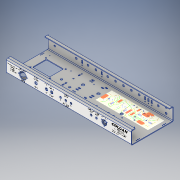
# Autodesk Inventor part: mainChassis
Saved by Autodesk Inventor 2018.1 (Build 221171000, 171)
## iProperties
Created: 2019-02-19
Part Number: mainChassis
Material: Aluminum 6061
Document SubType Name: Sheet Metal
Designer: RCCol
Density: 2.7 g/cm^3
Sheet Metal Rule: .125 thick aluminum
Appearance: Aluminum - Flat
Flat Pattern Width: 34.7497 cm
Flat Pattern Length: 60.325 cm
Flat Pattern Area: 2096.27 cm^2
Sheet Metal Width: 13.681 in
Sheet Metal Length: 23.750 in
Sheet Metal Area: 324.923 in^2
Author: RCCol
Autodesk Inventor part; units mm, degrees
ref_plane "YZ Plane" through (0, 0, 0) normal (1, 0, 0) x (0, 1, 0)
ref_plane "XZ Plane" through (0, 0, 0) normal (0, 1, 0) x (-1, 0, 0)
ref_plane "XY Plane" through (0, 0, 0) normal (0, 0, 1) x (1, 0, 0)
sketch "Sketch1" plane through (0, 0, 0) normal (0, 1, 0) x (-1, 0, 0)
  line L0 (0, 0) -> (-603.25, 0)
  line L1 (-603.25, 0) -> (-603.25, -204.47)
  line L2 (-603.25, -204.47) -> (0, -204.47)
  line L3 (0, -204.47) -> (0, 0)
  line L4 (0, 0) -> (-254, 0)
  line L5 (0, -79.375) -> (0, 0)
  dimension "d0" = 603.25
  dimension "d1" = 204.47
  constraints: 12 end point, 2 horizontal, 2 parallel, 1 perpendicular
  measures "d0" distance of L2.end L1.end
  measures "d1" distance of L1.end L0.end
extrude "Plate1" add sketch "Sketch1" along normal blind 3.175
sketch "Sketch2" plane through (0, 3.175, 0) normal (0, 1, 0) x (1, 0, 0)
  line L0 (41.3, 154.94) -> (117.45, 154.94)
  arc A0 (120.65, 151.74) -> (117.45, 154.94) centre (117.45, 151.74) ccw
  line L1 (41.3, 87.63) -> (117.45, 87.63)
  arc A1 (117.45, 87.63) -> (120.65, 90.83) centre (117.45, 90.83) ccw
  line L2 (38.1, 151.74) -> (38.1, 90.83)
  arc A2 (41.3, 154.94) -> (38.1, 151.74) centre (41.3, 151.74) ccw
  arc A3 (38.1, 90.83) -> (41.3, 87.63) centre (41.3, 90.83) ccw
  circle A4 centre (31.75, 177.5295) radius 1.5
  line L3 (120.65, 151.74) -> (120.65, 90.83)
  circle A5 centre (147.375, 75.2475) radius 1.65
  circle A6 centre (147.375, 164.1475) radius 1.65
  circle A7 centre (185.1575, 138.7475) radius 2.65
  circle A8 centre (185.1575, 178.435) radius 2.65
  circle A9 centre (235.9575, 87.1648) radius 2.65
  circle A10 centre (243.895, 87.1648) radius 2.65
  circle A11 centre (235.9575, 169.7148) radius 2.65
  circle A12 centre (243.895, 169.7148) radius 2.65
  circle A13 centre (259.135, 75.2475) radius 1.65
  circle A14 centre (355.6, 82.2325) radius 1.65
  circle A15 centre (259.135, 164.1475) radius 1.65
  circle A16 centre (355.6, 139.3825) radius 1.65
  circle A17 centre (536.575, 82.2325) radius 1.65
  circle A18 centre (536.575, 139.3825) radius 1.65
  arc A19 (187.6575, 169.4256) -> (182.6575, 169.4256) centre (185.1575, 169.4256) ccw
  arc A20 (182.6575, 164.4256) -> (187.6575, 164.4256) centre (185.1575, 164.4256) ccw
  line L4 (187.6575, 169.4256) -> (187.6575, 164.4256)
  line L5 (182.6575, 169.4256) -> (182.6575, 164.4256)
  arc A21 (187.6575, 90.4475) -> (182.6575, 90.4475) centre (185.1575, 90.4475) ccw
  arc A22 (182.6575, 85.4475) -> (187.6575, 85.4475) centre (185.1575, 85.4475) ccw
  line L6 (187.6575, 90.4475) -> (187.6575, 85.4475)
  line L7 (182.6575, 90.4475) -> (182.6575, 85.4475)
  arc A23 (308.1355, 175.935) -> (308.1355, 180.935) centre (308.1355, 178.435) ccw
  arc A24 (301.1355, 180.935) -> (301.1355, 175.935) centre (301.1355, 178.435) ccw
  line L8 (308.1355, 175.935) -> (301.1355, 175.935)
  line L9 (308.1355, 180.935) -> (301.1355, 180.935)
  arc A25 (243.048, 175.935) -> (243.048, 180.935) centre (243.048, 178.435) ccw
  arc A26 (236.048, 180.935) -> (236.048, 175.935) centre (236.048, 178.435) ccw
  line L10 (243.048, 175.935) -> (236.048, 175.935)
  line L11 (243.048, 180.935) -> (236.048, 180.935)
  arc A27 (298.195, 167.2148) -> (298.195, 172.2148) centre (298.195, 169.7148) ccw
  arc A28 (291.195, 172.2148) -> (291.195, 167.2148) centre (291.195, 169.7148) ccw
  line L12 (298.195, 167.2148) -> (291.195, 167.2148)
  line L13 (298.195, 172.2148) -> (291.195, 172.2148)
  arc A29 (308.1355, 110.435) -> (308.1355, 115.435) centre (308.1355, 112.935) ccw
  arc A30 (301.1355, 115.435) -> (301.1355, 110.435) centre (301.1355, 112.935) ccw
  line L14 (308.1355, 110.435) -> (301.1355, 110.435)
  line L15 (308.1355, 115.435) -> (301.1355, 115.435)
  arc A31 (308.1355, 99.735) -> (308.1355, 104.735) centre (308.1355, 102.235) ccw
  arc A32 (301.1355, 104.735) -> (301.1355, 99.735) centre (301.1355, 102.235) ccw
  line L16 (308.1355, 99.735) -> (301.1355, 99.735)
  line L17 (308.1355, 104.735) -> (301.1355, 104.735)
  arc A33 (243.048, 110.435) -> (243.048, 115.435) centre (243.048, 112.935) ccw
  arc A34 (236.048, 115.435) -> (236.048, 110.435) centre (236.048, 112.935) ccw
  line L18 (243.048, 110.435) -> (236.048, 110.435)
  line L19 (243.048, 115.435) -> (236.048, 115.435)
  arc A35 (243.048, 99.735) -> (243.048, 104.735) centre (243.048, 102.235) ccw
  arc A36 (236.048, 104.735) -> (236.048, 99.735) centre (236.048, 102.235) ccw
  line L20 (243.048, 99.735) -> (236.048, 99.735)
  line L21 (243.048, 104.735) -> (236.048, 104.735)
  arc A37 (298.195, 84.6648) -> (298.195, 89.6648) centre (298.195, 87.1648) ccw
  arc A38 (291.195, 89.6648) -> (291.195, 84.6648) centre (291.195, 87.1648) ccw
  line L22 (298.195, 84.6648) -> (291.195, 84.6648)
  line L23 (298.195, 89.6648) -> (291.195, 89.6648)
  circle A39 centre (237.6, 35.56) radius 15.1
  arc A40 (239.251, 57.4158) -> (238.6557, 58.0111) centre (238.6557, 57.4158) ccw
  arc A41 (238.6557, 53.1089) -> (239.251, 53.7042) centre (238.6557, 53.7042) ccw
  line L24 (239.251, 53.7042) -> (239.251, 57.4158)
  arc A42 (236.5443, 58.0111) -> (235.949, 57.4158) centre (236.5443, 57.4158) ccw
  line L25 (235.949, 53.7042) -> (235.949, 57.4158)
  line L26 (238.6557, 58.0111) -> (236.5443, 58.0111)
  line L27 (238.6557, 53.1089) -> (236.5443, 53.1089)
  arc A43 (235.949, 53.7042) -> (236.5443, 53.1089) centre (236.5443, 53.7042) ccw
  arc A44 (239.251, 17.4158) -> (238.6557, 18.0111) centre (238.6557, 17.4158) ccw
  arc A45 (238.6557, 13.1089) -> (239.251, 13.7042) centre (238.6557, 13.7042) ccw
  line L28 (239.251, 13.7042) -> (239.251, 17.4158)
  arc A46 (236.5443, 18.0111) -> (235.949, 17.4158) centre (236.5443, 17.4158) ccw
  line L29 (235.949, 13.7042) -> (235.949, 17.4158)
  line L30 (238.6557, 18.0111) -> (236.5443, 18.0111)
  line L31 (238.6557, 13.1089) -> (236.5443, 13.1089)
  arc A47 (235.949, 13.7042) -> (236.5443, 13.1089) centre (236.5443, 13.7042) ccw
  circle A48 centre (174.1, 35.56) radius 15.1
  arc A49 (175.751, 57.4158) -> (175.1557, 58.0111) centre (175.1557, 57.4158) ccw
  arc A50 (175.1557, 53.1089) -> (175.751, 53.7042) centre (175.1557, 53.7042) ccw
  line L32 (175.751, 53.7042) -> (175.751, 57.4158)
  arc A51 (173.0443, 58.0111) -> (172.449, 57.4158) centre (173.0443, 57.4158) ccw
  line L33 (172.449, 53.7042) -> (172.449, 57.4158)
  line L34 (175.1557, 58.0111) -> (173.0443, 58.0111)
  line L35 (175.1557, 53.1089) -> (173.0443, 53.1089)
  arc A52 (172.449, 53.7042) -> (173.0443, 53.1089) centre (173.0443, 53.7042) ccw
  arc A53 (175.751, 17.4158) -> (175.1557, 18.0111) centre (175.1557, 17.4158) ccw
  arc A54 (175.1557, 13.1089) -> (175.751, 13.7042) centre (175.1557, 13.7042) ccw
  line L36 (175.751, 13.7042) -> (175.751, 17.4158)
  arc A55 (173.0443, 18.0111) -> (172.449, 17.4158) centre (173.0443, 17.4158) ccw
  line L37 (172.449, 13.7042) -> (172.449, 17.4158)
  line L38 (175.1557, 18.0111) -> (173.0443, 18.0111)
  line L39 (175.1557, 13.1089) -> (173.0443, 13.1089)
  arc A56 (172.449, 13.7042) -> (173.0443, 13.1089) centre (173.0443, 13.7042) ccw
  circle A57 centre (110.6, 35.56) radius 15.1
  arc A58 (112.251, 57.4158) -> (111.6557, 58.0111) centre (111.6557, 57.4158) ccw
  arc A59 (111.6557, 53.1089) -> (112.251, 53.7042) centre (111.6557, 53.7042) ccw
  line L40 (112.251, 53.7042) -> (112.251, 57.4158)
  arc A60 (109.5443, 58.0111) -> (108.949, 57.4158) centre (109.5443, 57.4158) ccw
  line L41 (108.949, 53.7042) -> (108.949, 57.4158)
  line L42 (111.6557, 58.0111) -> (109.5443, 58.0111)
  line L43 (111.6557, 53.1089) -> (109.5443, 53.1089)
  arc A61 (108.949, 53.7042) -> (109.5443, 53.1089) centre (109.5443, 53.7042) ccw
  arc A62 (112.251, 17.4158) -> (111.6557, 18.0111) centre (111.6557, 17.4158) ccw
  arc A63 (111.6557, 13.1089) -> (112.251, 13.7042) centre (111.6557, 13.7042) ccw
  line L44 (112.251, 13.7042) -> (112.251, 17.4158)
  arc A64 (109.5443, 18.0111) -> (108.949, 17.4158) centre (109.5443, 17.4158) ccw
  line L45 (108.949, 13.7042) -> (108.949, 17.4158)
  line L46 (111.6557, 18.0111) -> (109.5443, 18.0111)
  line L47 (111.6557, 13.1089) -> (109.5443, 13.1089)
  arc A65 (108.949, 13.7042) -> (109.5443, 13.1089) centre (109.5443, 13.7042) ccw
  circle A66 centre (47.1, 35.56) radius 15.1
  arc A67 (48.751, 57.4158) -> (48.1557, 58.0111) centre (48.1557, 57.4158) ccw
  arc A68 (48.1557, 53.1089) -> (48.751, 53.7042) centre (48.1557, 53.7042) ccw
  line L48 (48.751, 53.7042) -> (48.751, 57.4158)
  arc A69 (46.0443, 58.0111) -> (45.449, 57.4158) centre (46.0443, 57.4158) ccw
  line L49 (45.449, 53.7042) -> (45.449, 57.4158)
  line L50 (48.1557, 58.0111) -> (46.0443, 58.0111)
  line L51 (48.1557, 53.1089) -> (46.0443, 53.1089)
  arc A70 (45.449, 53.7042) -> (46.0443, 53.1089) centre (46.0443, 53.7042) ccw
  arc A71 (48.751, 17.4158) -> (48.1557, 18.0111) centre (48.1557, 17.4158) ccw
  arc A72 (48.1557, 13.1089) -> (48.751, 13.7042) centre (48.1557, 13.7042) ccw
  line L52 (48.751, 13.7042) -> (48.751, 17.4158)
  arc A73 (46.0443, 18.0111) -> (45.449, 17.4158) centre (46.0443, 17.4158) ccw
  line L53 (45.449, 13.7042) -> (45.449, 17.4158)
  line L54 (48.1557, 18.0111) -> (46.0443, 18.0111)
  line L55 (48.1557, 13.1089) -> (46.0443, 13.1089)
  arc A74 (45.449, 13.7042) -> (46.0443, 13.1089) centre (46.0443, 13.7042) ccw
  circle A75 centre (159.7575, 106.3403) radius 4.8
  circle A76 centre (212.2, 93.5148) radius 4.8
  circle A77 centre (309.5568, 135.335) radius 6.35
  circle A78 centre (234.6268, 135.335) radius 6.35
  circle A79 centre (269.35, 26.9408) radius 1.651
  circle A80 centre (501.65, 37.1475) radius 9.525
  circle A81 centre (491.5472, 47.2503) radius 1.651
  circle A82 centre (511.7528, 27.0447) radius 1.651
  circle A83 centre (444.5, 37.1475) radius 9.525
  circle A84 centre (434.3972, 47.2503) radius 1.651
  circle A85 centre (454.6028, 27.0447) radius 1.651
  circle A86 centre (406.4, 37.1475) radius 9.525
  circle A87 centre (396.2972, 47.2503) radius 1.651
  circle A88 centre (416.5028, 27.0447) radius 1.651
  circle A89 centre (368.3, 37.1475) radius 9.525
  circle A90 centre (358.1972, 47.2503) radius 1.651
  circle A91 centre (378.4028, 27.0447) radius 1.651
  circle A92 centre (330.2, 37.1475) radius 9.525
  circle A93 centre (320.0972, 47.2503) radius 1.651
  circle A94 centre (340.3028, 27.0447) radius 1.651
  circle A95 centre (205.85, 26.9408) radius 1.651
  circle A96 centre (78.85, 26.9408) radius 1.651
  circle A97 centre (78.85, 63.0879) radius 1.651
  circle A98 centre (19.05, 63.0879) radius 1.651
  circle A99 centre (503.2375, 162.56) radius 1.651
  circle A100 centre (142.35, 26.035) radius 1.651
  circle A101 centre (22.225, 20.5908) radius 1.651
  arc A102 (187.6575, 104.4569) -> (182.6575, 104.4569) centre (185.1575, 104.4569) ccw
  arc A103 (182.6575, 99.4569) -> (187.6575, 99.4569) centre (185.1575, 99.4569) ccw
  line L56 (187.6575, 104.4569) -> (187.6575, 99.4569)
  line L57 (182.6575, 104.4569) -> (182.6575, 99.4569)
  circle A104 centre (458.7875, 172.085) radius 1.651
  circle A105 centre (193.85, 60.5908) radius 1.65
  circle A106 centre (217.85, 60.5908) radius 1.65
  circle A107 centre (205.85, 60.5908) radius 4.826
  circle A108 centre (257.35, 59.0033) radius 1.65
  circle A109 centre (281.35, 59.0033) radius 1.65
  circle A110 centre (269.35, 59.0033) radius 4.826
  circle A111 centre (137.16, 62.3578) radius 1.651
  circle A112 centre (522.2875, 162.56) radius 1.651
  circle A113 centre (477.8375, 172.085) radius 1.651
  circle A114 centre (491.2375, 172.085) radius 1.651
  circle A115 centre (445.3875, 172.085) radius 1.651
  circle A116 centre (438.15, 78.2625) radius 4.826
  circle A117 centre (412.75, 78.2625) radius 4.826
  circle A118 centre (467.3028, 92.3925) radius 2.3813
  circle A119 centre (506.908, 112.5724) radius 2.3813
  circle A120 centre (449.8015, 107.4686) radius 6.35
  circle A121 centre (494.6689, 127.4196) radius 2.3813
  circle A122 centre (368.3, 21.2725) radius 1.651
  circle A123 centre (501.65, 53.0225) radius 1.651
  circle A124 centre (406.4, 53.0225) radius 1.651
  circle A125 centre (368.3, 53.0225) radius 1.651
  circle A126 centre (31.75, 159.385) radius 3.175
  circle A127 centre (127, 159.385) radius 3.175
  circle A128 centre (31.75, 83.185) radius 3.175
  circle A129 centre (127, 83.185) radius 3.175
  circle A130 centre (539.75, 37.1475) radius 9.525
  circle A131 centre (529.6472, 47.2503) radius 1.651
  circle A132 centre (549.8528, 27.0447) radius 1.651
  circle A133 centre (539.75, 53.0225) radius 1.651
  circle A134 centre (78.85, 35.56) radius 3.2385
  circle A135 centre (142.35, 35.56) radius 3.2385
  circle A136 centre (205.85, 35.56) radius 3.2385
  circle A137 centre (269.35, 35.56) radius 3.2385
  circle A138 centre (6.35, 165.735) radius 2.667
  circle A139 centre (6.35, 158.3944) radius 1.5875
  circle A140 centre (6.35, 173.0756) radius 1.5875
  circle A141 centre (6.35, 38.735) radius 2.667
  circle A142 centre (6.35, 31.3944) radius 1.5875
  circle A143 centre (6.35, 46.0756) radius 1.5875
  circle A144 centre (596.9, 38.735) radius 2.667
  circle A145 centre (596.9, 46.0756) radius 1.5875
  circle A146 centre (596.9, 31.3944) radius 1.5875
  circle A147 centre (596.9, 165.735) radius 2.667
  circle A148 centre (596.9, 173.0756) radius 1.5875
  circle A149 centre (596.9, 158.3944) radius 1.5875
  circle A150 centre (288.4, 35.56) radius 3.2385
  circle A151 centre (117.45, 90.83) radius 3.2
  circle A152 centre (41.3, 90.83) radius 3.2
  circle A153 centre (41.3, 151.74) radius 3.2
  circle A154 centre (117.45, 151.74) radius 3.2
  line L58 (117.45, 87.63) -> (41.3, 87.63)
  line L59 (41.3, 87.63) -> (41.3, 154.94)
  line L60 (41.3, 154.94) -> (117.45, 154.94)
  line L61 (117.45, 154.94) -> (117.45, 87.63)
  line L62 (38.1, 90.83) -> (120.65, 90.83)
  line L63 (120.65, 90.83) -> (120.65, 151.74)
  line L64 (120.65, 151.74) -> (38.1, 151.74)
  line L65 (38.1, 151.74) -> (38.1, 90.83)
  constraints: 153 centre point, 132 end point, 116 point on circle, 4 coincident, 4 parallel, 2 horizontal, 2 horizontal alignment, 2 perpendicular, 2 point on line, 4 other
extrude "Cut1" cut sketch "Sketch2" against normal blind 3.175
sketch "Sketch3" plane through (603.25, 0, -3.175) normal (0, 0, 1) x (1, 0, 0)
  line L0 (-603.25, 0) -> (0, 0)
  line L1 (0, 0) -> (0, 63.5)
  line L2 (0, 63.5) -> (-603.25, 63.5)
  line L3 (-603.25, 63.5) -> (-603.25, 0)
  constraints: 6 end point, 1 horizontal, 1 perpendicular, 1 vertical
edge flange "Flange1" height 63.5 angle 90 thickness 3.175 bend radius 3.175 thickness toward (0, 0, 1) relief straight relief width 3.175 relief depth 1.5875 edges at (301.625, 3.175, 0) wall of the first edge with corners at (0, 0, -3.175) (603.25, 0, -3.175) (603.25, 63.5, -3.175) (0, 63.5, -3.175)
bend "Bend1"
corner "Corner1"
sketch "Sketch4" plane through (603.25, 60.325, 0) normal (0, 1, 0) x (-1, 0, 0)
  line L0 (603.25, 0) -> (0, 0)
  line L1 (0, 0) -> (0, -19.05)
  line L2 (0, -19.05) -> (603.25, -19.05)
  line L3 (603.25, -19.05) -> (603.25, 0)
  constraints: 6 end point, 1 horizontal, 1 perpendicular, 1 vertical
edge flange "Flange2" height 19.05 angle 90 thickness 3.175 bend radius 3.175 thickness toward (0, 1, 0) relief straight relief width 3.175 relief depth 1.5875 edges at (301.625, 63.5, -3.175) wall of the first edge with corners at (0, 60.325, 0) (603.25, 60.325, 0) (603.25, 60.325, -19.05) (0, 60.325, -19.05)
bend "Bend2"
corner "Corner2"
sketch "Sketch5" plane through (0, 6.35, 0) normal (0, 0, 1) x (1, 0, 0)
  circle A0 centre (78.85, 25.4) radius 17.4625
  circle A1 centre (99.805, 25.4) radius 1.778
  circle A2 centre (57.895, 25.4) radius 1.778
  line L0 (148.065, 22.0907) -> (148.065, 28.7093)
  line L1 (136.635, 22.0907) -> (136.635, 28.7093)
  arc A3 (136.635, 22.0907) -> (148.065, 22.0907) centre (142.35, 25.4) ccw
  arc A4 (148.065, 28.7093) -> (136.635, 28.7093) centre (142.35, 25.4) ccw
  line L2 (193.9018, 20.2386) -> (192.3982, 20.2386)
  arc A5 (193.9018, 19.2226) -> (192.3982, 19.2226) centre (193.15, 25.4) ccw
  line L3 (192.3982, 20.2386) -> (192.3982, 19.2226)
  line L4 (193.9018, 19.2226) -> (193.9018, 20.2386)
  line L5 (219.3018, 20.2386) -> (217.7982, 20.2386)
  arc A6 (219.3018, 19.2226) -> (217.7982, 19.2226) centre (218.55, 25.4) ccw
  line L6 (217.7982, 20.2386) -> (217.7982, 19.2226)
  line L7 (219.3018, 19.2226) -> (219.3018, 20.2386)
  circle A7 centre (261.3213, 25.4) radius 4.7625
  circle A8 centre (286.7213, 25.4) radius 4.7625
  circle A9 centre (312.1213, 25.4) radius 4.7625
  circle A10 centre (409.575, 25.5399) radius 4.7625
  circle A11 centre (434.975, 25.5399) radius 4.7625
  circle A12 centre (473.075, 25.5399) radius 12.1031
  circle A13 centre (460.2734, 32.9821) radius 1.778
  circle A14 centre (485.8766, 32.9821) radius 1.778
  circle A15 centre (473.075, 10.7317) radius 1.778
  line L8 (136.635, 28.7093) -> (148.065, 28.7093)
  line L9 (148.065, 28.7093) -> (148.065, 22.0907)
  line L10 (148.065, 22.0907) -> (136.635, 22.0907)
  line L11 (136.635, 22.0907) -> (136.635, 28.7093)
  arc A16 (148.065, 28.7093) -> (136.635, 28.7093) centre (142.35, 25.4) ccw
  arc A17 (136.635, 22.0907) -> (148.065, 22.0907) centre (142.35, 25.4) ccw
  arc A18 (136.635, 22.0907) -> (148.065, 22.0907) centre (142.35, 25.4) ccw
  arc A19 (193.9018, 19.2226) -> (192.3982, 19.2226) centre (193.15, 25.4) ccw
  line L12 (193.9018, 19.2226) -> (193.9018, 20.2386)
  line L13 (192.3982, 20.2386) -> (192.3982, 19.2226)
  point P0 (0, -6.35)
  constraints: 28 end point, 23 point on circle, 20 centre point, 5 point on line, 2 parallel, 1 concentric, 1 horizontal, 1 perpendicular, 1 vertical
extrude "Cut2" cut sketch "Sketch5" against normal blind 3.175
sketch "Sketch6" plane through (0, 0, -201.295) normal (0, 0, -1) x (-1, 0, 0)
  line L0 (-603.25, 0) -> (0, 0)
  line L1 (0, 0) -> (0, 63.5)
  line L2 (0, 63.5) -> (-603.25, 63.5)
  line L3 (-603.25, 63.5) -> (-603.25, 0)
  constraints: 6 end point, 1 horizontal, 1 perpendicular, 1 vertical
edge flange "Flange3" height 63.5 angle 90 thickness 3.175 bend radius 3.175 thickness toward (0, 0, -1) relief straight relief width 3.175 relief depth 1.5875 edges at (301.625, 3.175, -204.47) wall of the first edge with corners at (603.25, 0, -201.295) (0, 0, -201.295) (0, 63.5, -201.295) (603.25, 63.5, -201.295)
bend "Bend3"
corner "Corner3"
sketch "Sketch7" plane through (0, 60.325, -204.47) normal (0, 1, 0) x (-1, 0, 0)
  line L0 (-603.25, 0) -> (0, 0)
  line L1 (0, 0) -> (0, 19.05)
  line L2 (0, 19.05) -> (-603.25, 19.05)
  line L3 (-603.25, 19.05) -> (-603.25, 0)
  constraints: 6 end point, 1 horizontal, 1 perpendicular, 1 vertical
edge flange "Flange4" height 19.05 angle 90 thickness 3.175 bend radius 3.175 thickness toward (0, 1, 0) relief straight relief width 3.175 relief depth 1.5875 edges at (301.625, 63.5, -201.295) wall of the first edge with corners at (603.25, 60.325, -204.47) (0, 60.325, -204.47) (0, 60.325, -185.42) (603.25, 60.325, -185.42)
bend "Bend4"
corner "Corner4"
sketch "Sketch8" plane through (603.25, 6.35, -204.47) normal (0, 0, -1) x (-1, 0, 0)
  circle A0 centre (31.9541, 38.1) radius 4.7625
  circle A1 centre (70.0541, 25.4) radius 4.7625
  circle A2 centre (200.4831, 25.4) radius 4.7625
  circle A3 centre (314.7831, 25.4) radius 4.7625
  circle A4 centre (467.1831, 25.4) radius 4.7625
  circle A5 centre (410.0331, 25.4) radius 4.7625
  circle A6 centre (371.9331, 25.4) radius 4.7625
  circle A7 centre (276.6831, 25.4) radius 4.7625
  circle A8 centre (238.5831, 25.4) radius 4.7625
  circle A9 centre (162.3831, 25.4) radius 4.7625
  circle A10 centre (31.9541, 12.7) radius 4.7625
  circle A11 centre (31.9541, 12.7) radius 4.7625
  circle A12 centre (162.3831, 25.4) radius 4.7625
  circle A13 centre (238.5831, 25.4) radius 4.7625
  circle A14 centre (276.6831, 25.4) radius 4.7625
  circle A15 centre (371.9331, 25.4) radius 4.7625
  circle A16 centre (410.0331, 25.4) radius 4.7625
  circle A17 centre (467.1831, 25.4) radius 4.7625
  circle A18 centre (314.7831, 25.4) radius 4.7625
  circle A19 centre (200.4831, 25.4) radius 4.7625
  circle A20 centre (70.0541, 25.4) radius 4.7625
  circle A21 centre (31.9541, 38.1) radius 4.7625
  circle A22 centre (571.5, 25.4) radius 3.9624
  circle A23 centre (101.8041, 39.6875) radius 1.9558
  circle A24 centre (101.8041, 11.1125) radius 1.9558
  line L0 (98.6291, 31.75) -> (104.9791, 31.75)
  line L1 (104.9791, 31.75) -> (104.9791, 19.05)
  line L2 (104.9791, 19.05) -> (98.6291, 19.05)
  line L3 (98.6291, 19.05) -> (98.6291, 31.75)
  circle A25 centre (117.8061, 39.6875) radius 1.9558
  circle A26 centre (117.8061, 11.1125) radius 1.9558
  line L4 (114.6311, 31.75) -> (120.9811, 31.75)
  line L5 (120.9811, 31.75) -> (120.9811, 19.05)
  line L6 (120.9811, 19.05) -> (114.6311, 19.05)
  line L7 (114.6311, 19.05) -> (114.6311, 31.75)
  circle A27 centre (133.8081, 39.6875) radius 1.9558
  circle A28 centre (133.8081, 11.1125) radius 1.9558
  line L8 (130.6331, 31.75) -> (136.9831, 31.75)
  line L9 (136.9831, 31.75) -> (136.9831, 19.05)
  line L10 (136.9831, 19.05) -> (130.6331, 19.05)
  line L11 (130.6331, 19.05) -> (130.6331, 31.75)
  circle A29 centre (343.3581, 39.6875) radius 1.9558
  circle A30 centre (343.3581, 11.1125) radius 1.9558
  line L12 (340.1831, 31.75) -> (346.5331, 31.75)
  line L13 (346.5331, 31.75) -> (346.5331, 19.05)
  line L14 (346.5331, 19.05) -> (340.1831, 19.05)
  line L15 (340.1831, 19.05) -> (340.1831, 31.75)
  circle A31 centre (438.6081, 39.6875) radius 1.9558
  circle A32 centre (438.6081, 11.1125) radius 1.9558
  line L16 (435.4331, 31.75) -> (441.7831, 31.75)
  line L17 (441.7831, 31.75) -> (441.7831, 19.05)
  line L18 (441.7831, 19.05) -> (435.4331, 19.05)
  line L19 (435.4331, 19.05) -> (435.4331, 31.75)
  line L20 (98.6291, 31.75) -> (104.9791, 31.75)
  line L21 (104.9791, 31.75) -> (104.9791, 19.05)
  line L22 (104.9791, 19.05) -> (98.6291, 19.05)
  line L23 (98.6291, 19.05) -> (98.6291, 31.75)
  line L24 (114.6311, 31.75) -> (120.9811, 31.75)
  line L25 (120.9811, 31.75) -> (120.9811, 19.05)
  line L26 (120.9811, 19.05) -> (114.6311, 19.05)
  line L27 (114.6311, 19.05) -> (114.6311, 31.75)
  line L28 (130.6331, 31.75) -> (136.9831, 31.75)
  line L29 (136.9831, 31.75) -> (136.9831, 19.05)
  line L30 (136.9831, 19.05) -> (130.6331, 19.05)
  line L31 (130.6331, 19.05) -> (130.6331, 31.75)
  line L32 (441.7831, 31.75) -> (435.4331, 31.75)
  line L33 (435.4331, 31.75) -> (435.4331, 19.05)
  line L34 (435.4331, 19.05) -> (441.7831, 19.05)
  line L35 (441.7831, 19.05) -> (441.7831, 31.75)
  line L36 (346.5331, 31.75) -> (340.1831, 31.75)
  line L37 (340.1831, 31.75) -> (340.1831, 19.05)
  line L38 (340.1831, 19.05) -> (346.5331, 19.05)
  line L39 (346.5331, 19.05) -> (346.5331, 31.75)
  constraints: 80 end point, 33 centre point, 10 parallel, 5 horizontal, 5 perpendicular
extrude "Cut3" cut sketch "Sketch8" against normal blind 3.175
sketch "Sketch9" plane through (603.25, 6.35, -204.47) normal (0, 0, -1) x (-1, 0, 0)
  line L0 (0, 50.8) -> (0, 53.975) projected
  line L1 (0, 53.975) -> (603.25, 53.975) projected
  line L2 (603.25, 53.975) -> (0, 53.975) projected
  line L3 (0, 53.975) -> (603.2512, 53.975) construction
  line L4 (603.2512, 53.975) -> (603.2512, -3.1751) construction
  line L5 (603.2512, -3.1751) -> (0, -3.1751) construction
  line L6 (0, -3.1751) -> (0, 53.975) construction
  point P0 (603.25, -6.35)
  constraints: 2 other
decal "Decal1"
sketch "Sketch10" plane through (0, 6.35, 0) normal (0, 0, 1) x (1, 0, 0)
  line L0 (0, 53.975) -> (603.2512, 53.975) construction
  line L1 (603.2512, 53.975) -> (603.2512, -3.1751) construction
  line L2 (603.2512, -3.1751) -> (0, -3.1751) construction
  line L3 (0, -3.1751) -> (0, 53.975) construction
  point P0 (0, -6.35)
  constraints: 2 other
decal "Decal2"
sketch "Sketch11" plane through (0, 3.175, 0) normal (0, 1, 0) x (1, 0, 0)
  line L0 (327.7837, 182.0084) -> (581.4999, 182.0084) construction
  line L1 (581.4999, 182.0084) -> (581.4999, 102.7644) construction
  line L2 (581.4999, 102.7644) -> (327.7837, 102.7644) construction
  line L3 (327.7837, 102.7644) -> (327.7837, 182.0084) construction
  point P0 (0, 0)
  constraints: 2 other
decal "Decal3"
equation "\"d3\" = Thickness"
equation "\"d27\" = Thickness"
equation "\"d49\" = Thickness"
equation "\"d2\" = Thickness"
equation "\"d5\" = BendReliefWidth"
equation "\"d6\" = BendReliefDepth"
equation "\"d7\" = MinimumRemnant"
equation "\"d8\" = TransitionRadius"
equation "\"d11\" = BendRadius"
equation "\"d12\" = CornerReliefSize"
equation "\"d13\" = GapSize"
equation "\"d14\" = JacobiRadiusSize"
equation "\"d17\" = BendReliefWidth"
equation "\"d18\" = BendReliefDepth"
equation "\"d19\" = MinimumRemnant"
equation "\"d20\" = TransitionRadius"
equation "\"d23\" = BendRadius"
equation "\"d24\" = CornerReliefSize"
equation "\"d25\" = GapSize"
equation "\"d26\" = JacobiRadiusSize"
equation "\"d29\" = BendReliefWidth"
equation "\"d30\" = BendReliefDepth"
equation "\"d31\" = MinimumRemnant"
equation "\"d32\" = TransitionRadius"
equation "\"d35\" = BendRadius"
equation "\"d36\" = CornerReliefSize"
equation "\"d37\" = GapSize"
equation "\"d38\" = JacobiRadiusSize"
equation "\"d39\" = BendReliefWidth"
equation "\"d40\" = BendReliefDepth"
equation "\"d41\" = MinimumRemnant"
equation "\"d42\" = TransitionRadius"
equation "\"d45\" = BendRadius"
equation "\"d46\" = CornerReliefSize"
equation "\"d47\" = GapSize"
equation "\"d48\" = JacobiRadiusSize"
equation "\"BendRadius\" = Thickness"
equation "\"BendReliefWidth\" = Thickness"
equation "\"BendReliefDepth\" = 0.5 * Thickness"
equation "\"CornerReliefSize\" = 4 * Thickness"
equation "\"MinimumRemnant\" = 2 * Thickness"
equation "\"TransitionRadius\" = BendRadius"
equation "\"JacobiRadiusSize\" = BendRadius"
equation "\"GapSize\" = Thickness"
equation "\"Thickness\" = 3.175"
body "Solid1"
